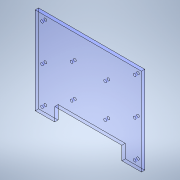
# Autodesk Inventor part: Plaque avant
Saved by Autodesk Inventor 2022 (Build 260153000, 153)
## iProperties
Created: 2022-05-23
Part Number: Plaque avant
Material: Générique
Document SubType Name: Modeling
Designer: victo
Density: 1 g/cm^3
Appearance: Transparent - Bleu
Author: victo
Autodesk Inventor part; units mm, degrees
ref_plane "YZ Plane" through (0, 0, 0) normal (1, 0, 0) x (0, 1, 0)
ref_plane "XZ Plane" through (0, 0, 0) normal (0, 1, 0) x (-1, 0, 0)
ref_plane "XY Plane" through (0, 0, 0) normal (0, 0, 1) x (1, 0, 0)
sketch "Esquisse1" plane through (0, 0, 0) normal (0, 0, 1) x (1, 0, 0)
  line L0 (0, 0) -> (-50, 0)
  line L1 (-50, 0) -> (-50, -20)
  line L2 (-50, -20) -> (-79, -20)
  line L3 (-79, -20) -> (-79, 110)
  line L4 (-79, 110) -> (79, 110)
  line L5 (79, 110) -> (79, -20)
  line L6 (79, -20) -> (50, -20)
  line L7 (50, -20) -> (50, 0)
  line L8 (50, 0) -> (0, 0)
  line L9 (-69, 110) -> (-69, 100)
  line L10 (-69, 100) -> (-69, 45) construction
  line L11 (-69, 45) -> (-69, -10) construction
  line L12 (-69, -10) -> (-69, -20)
  line L13 (69, -20) -> (69, -10)
  line L14 (69, -10) -> (69, 45) construction
  line L15 (69, 45) -> (69, 100) construction
  line L16 (69, 100) -> (69, 110)
  circle A0 centre (-69, 100) radius 2
  circle A1 centre (69, 100) radius 2
  circle A2 centre (69, 45) radius 2
  circle A3 centre (-69, 45) radius 2
  circle A4 centre (-69, -10) radius 2
  circle A5 centre (69, -10) radius 2
  line L17 (-69, -10) -> (-79, -10)
  line L18 (69, -10) -> (79, -10)
  line L19 (25, 70) -> (-25, 70) construction
  line L20 (-25, 70) -> (-25, 20) construction
  line L21 (-25, 20) -> (25, 20) construction
  line L22 (25, 20) -> (25, 70) construction
  line L23 (25, 70) -> (-25, 20) construction
  line L24 (-25, 70) -> (25, 20) construction
  line L25 (-69, 45) -> (69, 45) construction
  circle A6 centre (-25, 70) radius 2
  circle A7 centre (25, 70) radius 2
  circle A8 centre (25, 20) radius 2
  circle A9 centre (-25, 20) radius 2
  point P0 (0, 45)
  dimension "d0" = 130
  dimension "d1" = 110
  dimension "d2" = 100
  dimension "d3" = 158
  dimension "d4" = 10
  dimension "d5" = 4
  dimension "d8" = 4
  dimension "d9" = 50
  dimension "d10" = 50
  constraints: 52 end point, 14 point on line, 10 centre point, 10 equal length, 10 perpendicular, 9 coincident, 8 equal radius, 3 horizontal, 3 midpoint, 2 parallel, 2 vertical
  measures "d0" distance between parallel lines of L2 L4
  measures "d1" distance between parallel lines of L4 L0
  measures "d2" distance between parallel lines of L1 L7
  measures "d3" distance between parallel lines of L3 L5
  measures "d4" distance of L9.start L9.end
  measures "d5" diameter of A3
  measures "d8" diameter of A9
  measures "d9" distance of L19.end L20.end
  measures "d10" distance of L19.start L19.end
extrude "Extrusion1" add sketch "Esquisse1" against normal blind 5 contours L0 L1 L2 L12 A4 L17 L3 L4 L5 L18 A5 L13 L6 L7 L8 | L2 L3 L17 A4 L12 | L13 A5 L18 L5 L6
